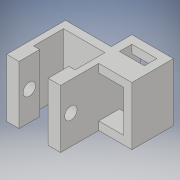
# Autodesk Inventor part: Frame_Clamp
Saved by Autodesk Inventor 2019 (Build 230136000, 136)
## iProperties
Created: 2019-10-14
Part Number: Frame_Clamp
Material: Generic
Document SubType Name: Modeling
Designer: James
Density: 1 g/cm^3
Appearance: Default
Author: James
Autodesk Inventor part; units mm, degrees
ref_plane "YZ Plane" through (0, 0, 0) normal (1, 0, 0) x (0, 1, 0)
ref_plane "XZ Plane" through (0, 0, 0) normal (0, 1, 0) x (-1, 0, 0)
ref_plane "XY Plane" through (0, 0, 0) normal (0, 0, 1) x (1, 0, 0)
sketch "Sketch1" plane through (0, 0, 0) normal (0, 1, 0) x (-1, 0, 0)
  line L0 (5, 3.6) -> (-5, 3.6)
  line L1 (-5, 3.6) -> (-5, -3.6)
  line L2 (-5, -3.6) -> (5, -3.6)
  line L3 (5, -3.6) -> (5, 3.6)
  line L4 (6.5, 8.6) -> (6.5, -5.6)
  line L5 (6.5, -5.6) -> (-6.5, -5.6)
  line L6 (-6.5, -5.6) -> (-6.5, 8.6)
  line L7 (-6.5, 8.6) -> (-3.5, 8.6)
  line L8 (6.5, 8.6) -> (3.5, 8.6)
  line L9 (3.5, 8.6) -> (3.5, 3.6)
  line L10 (-3.5, 8.6) -> (-3.5, 3.6)
  point P0 (0, 0)
  point P1 (5, 0)
  point P2 (0, -3.6)
  point P3 (-5, 8.6)
  point P4 (5, 8.6)
  dimension "d0" = 7.2
  dimension "d1" = 10
  dimension "d2" = 1.5
  dimension "d3" = 1.5
  dimension "d4" = 5
  dimension "d5" = 1.5
  dimension "d6" = 2
  constraints: 22 end point, 6 perpendicular, 4 midpoint, 3 horizontal, 2 horizontal alignment, 2 parallel, 2 point on line, 1 collinear, 1 vertical alignment
  measures "d0" distance of L0.end L1.end
  measures "d1" distance of L1.end L2.end
  measures "d2" distance between parallel lines of L4 L3
  measures "d3" distance between parallel lines of L6 L1
  measures "d4" distance between parallel lines of L0 L8
  measures "d5" distance between parallel lines of L3 L9
  measures "d6" distance between parallel lines of L5 L2
extrude "Extrusion1" add sketch "Sketch1" along normal blind 14 contours L0 L9 L8 L4 L5 L6 L7 L10 L1 L2 L3
sketch "Sketch2" plane through (6.5, 0, 8.6) normal (1, 0, 0) x (0, 0, -1)
  circle A0 centre (2.5, 7) radius 1.5
  line L0 (0, 0) -> (0, 14) projected
  point P0 (8.6, 0)
  point P1 (0, 7)
  dimension "d9" = 2.5
  dimension "d10" = 3
  constraints: 1 centre point, 1 horizontal alignment, 1 midpoint
  measures "d9" distance from line of L0 A0.centre
  measures "d10" diameter of A0
extrude "Extrusion2" cut sketch "Sketch2" against normal blind 14.75
sketch "Sketch3" plane through (6.5, 0, -5.6) normal (0, 0, -1) x (-1, 0, 0)
  line L0 (3, 0) -> (0, 0) projected
  line L1 (0, 0) -> (-6, 0)
  line L2 (-6, 0) -> (-6, 2)
  line L3 (-6, 2) -> (0, 2)
  line L4 (0, 2) -> (0, 0)
  line L5 (3, 14) -> (0, 14) projected
  line L6 (0, 14) -> (-6, 14)
  line L7 (-6, 14) -> (-6, 12)
  line L8 (-6, 12) -> (0, 12)
  line L9 (0, 12) -> (0, 14)
  line L10 (0, 0) -> (0, 14) projected
  point P0 (6.5, 0)
  point P1 (-6, 1)
  point P2 (-6, 13)
  dimension "d13" = 2
  dimension "d14" = 2
  dimension "d15" = 6
  constraints: 16 end point, 4 parallel, 2 horizontal, 2 midpoint, 2 perpendicular, 1 vertical alignment
  measures "d13" distance of L1.end L2.end
  measures "d14" distance of L6.end L7.end
  measures "d15" distance between parallel lines of L10 L2
extrude "Extrusion3" add sketch "Sketch3" along normal mid plane 10
sketch "Sketch4" plane through (-6.5, 0, -5.6) normal (0, 0, -1) x (-1, 0, 0)
  line L0 (-13, 0) -> (-13, 14) projected
  line L1 (-10, 0) -> (-13, 0) projected
  line L2 (-13, 14) -> (-11, 14)
  line L3 (-11, 14) -> (-11, 0)
  line L4 (-11, 0) -> (-13, 0)
  line L5 (-13, 0) -> (-13, 14)
  point P0 (-6.5, 0)
  dimension "d18" = 2
  constraints: 8 end point, 2 parallel, 1 horizontal, 1 perpendicular, 1 point on line
  measures "d18" distance between parallel lines of L0 L3
extrude "Extrusion4" add sketch "Sketch4" along normal blind 5
sketch "Sketch5" plane through (0, 0, 0) normal (0, -1, 0) x (1, 0, 0)
  line L0 (12.5, -0.6) -> (12.5, -10.6) projected
  line L1 (6.5, -0.6) -> (6.5, -10.6) projected
  line L2 (12.5, -8.6) -> (6.5, -8.6)
  line L3 (6.5, -8.6) -> (6.5, -5.6)
  line L4 (6.5, -5.6) -> (12.5, -5.6)
  line L5 (12.5, -5.6) -> (12.5, -8.6)
  point P0 (0, 0)
  point P1 (9.5, -5.6)
  point P2 (4.5, -5.6)
  dimension "d21" = 3
  constraints: 8 end point, 2 midpoint, 2 parallel, 1 horizontal, 1 horizontal alignment, 1 perpendicular, 1 point on line
  measures "d21" distance between parallel lines of L2 L4
extrude "Extrusion5" cut sketch "Sketch5" against normal blind 23.5
sketch "Sketch6" plane through (12.5, 0, -0.6) normal (1, 0, 0) x (0, 0, -1)
  line L0 (0, 0) -> (0, 2) projected
  line L1 (8, 14) -> (10, 14) projected
  line L2 (0, 0) -> (10, 0)
  line L3 (10, 0) -> (10, 14)
  line L4 (10, 14) -> (0, 14)
  line L5 (0, 14) -> (0, 0)
  point P0 (-0.6, 0)
  constraints: 8 end point, 2 parallel, 1 horizontal, 1 perpendicular
extrude "Extrusion6" add sketch "Sketch6" along normal blind 2
body "Solid1"
